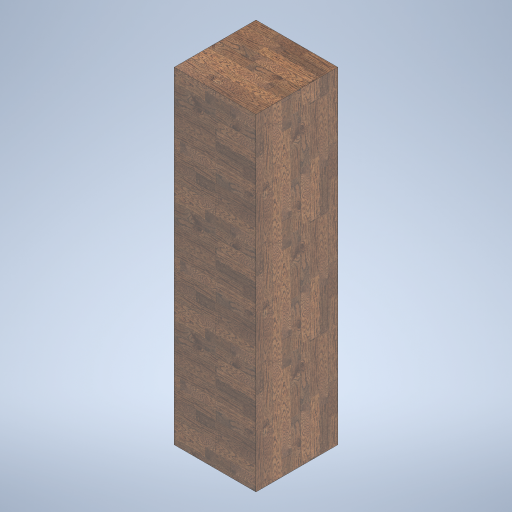
# Autodesk Inventor part: pillarofdeck
Saved by Autodesk Inventor 2023 (Build 270158000, 158)
## iProperties
Created: 2023-10-23
Part Number: pillarofdeck
Material: Wood (Oak)
Document SubType Name: Modeling
Designer: student
Density: 0.76 g/cm^3
Appearance: White Ash - Java
Author: student
Autodesk Inventor part; units mm, degrees
ref_plane "YZ Plane" through (0, 0, 0) normal (1, 0, 0) x (0, 1, 0)
ref_plane "XZ Plane" through (0, 0, 0) normal (0, 1, 0) x (-1, 0, 0)
ref_plane "XY Plane" through (0, 0, 0) normal (0, 0, 1) x (1, 0, 0)
sketch "Sketch1" plane through (0, 0, 0) normal (0, 0, 1) x (1, 0, 0)
  line L0 (0, 0) -> (500, 0)
  line L1 (500, 0) -> (500, 2000)
  line L2 (500, 2000) -> (0, 2000)
  line L3 (0, 2000) -> (0, 0)
  dimension "d0" = 2000
  dimension "d1" = 500
  constraints: 8 end point, 2 parallel, 1 horizontal, 1 perpendicular
  measures "d0" distance of L0.end L1.end
  measures "d1" distance of L1.end L2.end
extrude "Extrusion1" add sketch "Sketch1" along normal blind 500
body "Solid1"
